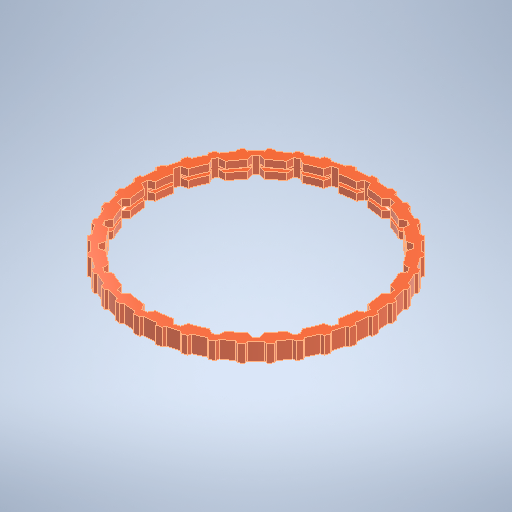
# Autodesk Inventor part: 3D_TPU-cover
Saved by Autodesk Inventor 2025 (Build 290162000, 162)
## iProperties
Created: 2024-07-17
Part Number: 3D_TPU-cover
Material: 一般
Document SubType Name: Modeling
Designer: 8326d
Density: 1 g/cm^3
Appearance: 滑らか - 淡いオレンジ
Author: 8326d
## iProperties of the stored document 3D_TPU-cover_3D プリント.ipt
Created: 2024-07-27
Part Number: 3D_TPU-cover_3D プリント
Material: 一般
Document SubType Name: Modeling
Designer: 8326d
Density: 1 g/cm^3
Appearance: 既定
Author: 8326d
Autodesk Inventor part; units mm, degrees
ref_plane "YZ Plane" through (0, 0, 0) normal (1, 0, 0) x (0, 1, 0)
ref_plane "XZ Plane" through (0, 0, 0) normal (0, 1, 0) x (-1, 0, 0)
ref_plane "XY Plane" through (0, 0, 0) normal (0, 0, 1) x (1, 0, 0)
sketch "スケッチ1" plane through (0, 0, 0) normal (0, 1, 0) x (-1, 0, 0)
  circle A0 centre (0, 0) radius 44
  circle A1 centre (0, 0) radius 40
  dimension "d0" = 88
  dimension "d1" = 80
  constraints: 2 centre point, 2 coincident
  measures "d0" diameter of A0
  measures "d1" diameter of A1
extrude "押し出し1" add sketch "スケッチ1" along normal mid plane 6.4
sketch "スケッチ2" plane through (0, 0, 0) normal (0, 1, 0) x (-1, 0, 0)
  circle A0 centre (0, 0) radius 40 projected
  circle A1 centre (0, 0) radius 42
  line L0 (0, 0) -> (42, 0) construction
  line L1 (0, 0) -> (40.5689, -10.8704) construction
  line L2 (0, 0) -> (42, 0) construction
  line L3 (39.9404, -2.1822) -> (41.9881, -1)
  line L4 (39.1443, -8.2295) -> (40.8162, -9.9014)
  dimension "d4" = 84
  dimension "d5" = 15
  dimension "d6" = 30
  dimension "d7" = 30
  dimension "d8" = 1
  dimension "d9" = 1
  constraints: 10 end point, 6 point on circle, 2 horizontal, 1 centre point, 1 coincident, 1 equal length
  measures "d4" diameter of A1
  measures "d5" angle of L1 L2
  measures "d6" angle of L0 L3
  measures "d7" angle of L1 L4
  measures "d8" distance from line of L0 L3.end
  measures "d9" distance from line of L1 L4.end
extrude "押し出し2" cut sketch "スケッチ2" along normal mid plane 1.2 contours A0 L3 A1 L4 picked at (40.9135, -5.7284)
chamfer "面取り1" distance 0.4 angle 45 2 edges at (-41.6407, -0.6, -5.4821) (-41.6407, 0.6, -5.4821)
sketch "スケッチ3" plane through (0, 3.2, 0) normal (0, 1, 0) x (1, 0, 0)
  circle A0 centre (0, 0) radius 42
  circle A1 centre (0, 0) radius 44 projected
  circle A2 centre (0, 0) radius 40 projected
  line L0 (-42, 0) -> (-40, 0)
  arc A3 (-40.4844, 9.5696) -> (-41.5817, 1.2346) centre (0, 0) ccw projected
  line L1 (0, 0) -> (-40.5689, 10.8704)
  line L2 (0, 0) -> (42, 0) construction
  line L3 (-41.5817, 1.2346) -> (-39.9404, 2.1822) projected
  line L4 (-39.1443, 8.2295) -> (-40.4844, 9.5696) projected
  line L5 (-41.5817, 1.2346) -> (-41.9881, 1)
  line L6 (-40.4844, 9.5696) -> (-40.8162, 9.9014)
  point P0 (-38.637, 10.3528)
  dimension "d15" = 84
  dimension "d16" = 165
  constraints: 10 end point, 5 point on circle, 2 collinear, 2 horizontal, 1 centre point, 1 coincident, 1 equal length, 1 horizontal alignment
  measures "d15" diameter of A0
  measures "d16" angle of L2 L1
extrude "押し出し3" cut sketch "スケッチ3" against normal through all contours L1 A2 L4 L6 A0 | A0 L5 L3 A2 L0
pattern_circular "円形状パターン1" count 24 over 360 about axis through (0, -10, 0) along (0, 1, 0) of "押し出し2", "面取り1", "押し出し3"
sketch "スケッチ4" plane through (0, 3.2, 0) normal (0, 1, 0) x (1, 0, 0)
  circle A0 centre (0, 0) radius 44 projected
  line L0 (-1.5875, 43.9714) -> (-1, 44.9889)
  line L1 (1.5875, 43.9714) -> (1, 44.9889)
  arc A1 (1, 44.9889) -> (-1, 44.9889) centre (0, 0) ccw
  line L2 (0, 44) -> (0, 0) construction
  point P0 (0, 45)
  dimension "d22" = 30
  dimension "d23" = 30
  dimension "d25" = 45
  dimension "d26" = 2
  constraints: 7 end point, 6 point on circle, 1 centre point, 1 coincident, 1 line through centre, 1 vertical, 1 vertical alignment
  measures "d22" angle of L2 L0
  measures "d23" angle of L2 L1
  measures "d25" radius of A1
  measures "d26" distance of L1.end L0.end
extrude "押し出し4" add sketch "スケッチ4" against normal up to surface (6.4 mm away) contours A0 L0 A1 L1
pattern_circular "円形状パターン2" count 36 over 360 about axis through (0, -10, 0) along (0, 1, 0) of "押し出し4"
equation "\"d7\" = d6"
equation "\"d9\" = d8"
equation "\"d23\" = d22"
